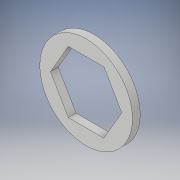
# Autodesk Inventor part: 0.0625 Hex Spacer
Saved by Autodesk Inventor 2018 (Build 220112000, 112)
## iProperties
Created: 2020-01-28
Part Number: 0.0625 Hex Spacer
Material: Generic
Document SubType Name: Modeling
Designer: maste
Density: 1 g/cm^3
Appearance: Default
Author: maste
Autodesk Inventor part; units mm, degrees
ref_plane "YZ Plane" through (0, 0, 0) normal (1, 0, 0) x (0, 1, 0)
ref_plane "XZ Plane" through (0, 0, 0) normal (0, 1, 0) x (-1, 0, 0)
ref_plane "XY Plane" through (0, 0, 0) normal (0, 0, 1) x (1, 0, 0)
sketch "Sketch1" plane through (0, 0, 0) normal (0, 0, 1) x (1, 0, 0)
  line L0 (7.3323, 0) -> (3.6662, -6.35)
  line L1 (3.6662, -6.35) -> (-3.6662, -6.35)
  line L2 (-3.6662, -6.35) -> (-7.3323, 0)
  line L3 (-7.3323, 0) -> (-3.6662, 6.35)
  line L4 (-3.6662, 6.35) -> (3.6662, 6.35)
  line L5 (3.6662, 6.35) -> (7.3323, 0)
  circle A0 centre (0, 0) radius 9.525
  dimension "d0" = 12.7
  dimension "d1" = 19.05
  constraints: 12 end point, 2 coincident, 1 centre point, 13 other
  measures "d0" distance between parallel lines of L1 L4
  measures "d1" diameter of A0
extrude "Extrusion1" add sketch "Sketch1" along normal blind 1.5875
body "Solid1"
